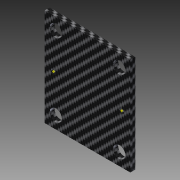
# Autodesk Inventor part: carbon_bump_servo
Saved by Autodesk Inventor 2015 SP1 (Build 190203100, 203)
## iProperties
Created: 2015-07-16
Part Number: carbon_bump_servo
Material: Generic
Document SubType Name: Modeling
Designer: Alexandre Cherpillod
Density: 1 g/cm^3
Appearance: Carbon Fiber
Mass: 2.63035 g
Surface Area: 30.8115 cm^2
Volume: 2.63035 cm^3
Author: Alexandre Cherpillod
Autodesk Inventor part; units mm, degrees
ref_plane "YZ Plane" through (0, 0, 0) normal (1, 0, 0) x (0, 1, 0)
ref_plane "XZ Plane" through (0, 0, 0) normal (0, 1, 0) x (-1, 0, 0)
ref_plane "XY Plane" through (0, 0, 0) normal (0, 0, 1) x (1, 0, 0)
sketch "Sketch1" plane through (0, 0, 0) normal (0, 1, 0) x (-1, 0, 0)
  line L0 (0, 0) -> (35, 0)
  line L1 (35, 0) -> (35, -40)
  line L2 (35, -40) -> (0, -40)
  line L3 (0, -40) -> (0, 0)
  line L4 (35, -40) -> (0, 0) construction
  line L5 (35, 0) -> (0, -40) construction
  line L6 (4.5, -5) -> (30.5, -5) construction
  line L7 (30.5, -5) -> (30.5, -35) construction
  line L8 (30.5, -35) -> (4.5, -35) construction
  line L9 (4.5, -35) -> (4.5, -5) construction
  line L10 (4.5, -5) -> (30.5, -35) construction
  line L11 (30.5, -5) -> (4.5, -35) construction
  circle A0 centre (30.5, -5) radius 2.5
  circle A1 centre (30.5, -35) radius 2.5
  circle A2 centre (4.5, -35) radius 2.5
  circle A3 centre (4.5, -5) radius 2.5
  point P0 (17.5, -20)
  dimension "d0" = 35
  dimension "d1" = 40
  dimension "d2" = 26
  dimension "d3" = 30
  dimension "d4" = 5
  constraints: 24 end point, 4 centre point, 4 coincident, 4 parallel, 3 equal radius, 3 midpoint, 2 horizontal, 2 perpendicular
  measures "d0" distance of L1.end L2.end
  measures "d1" distance of L0.end L1.end
  measures "d2" distance of L7.end L8.end
  measures "d3" distance of L6.end L7.end
  measures "d4" diameter of A0
extrude "Extrusion1" add sketch "Sketch1" along normal blind 2
sketch "Sketch2" plane through (0, 0, 0) normal (0, -1, 0) x (1, 0, 0)
  line L0 (-47.1371, -20) -> (16.7906, -20) construction
  line L1 (-30.5, -5) -> (-4.5, -35) construction
  line L2 (-4.5, -5) -> (-30.5, -35) construction
  point P0 (0, 0)
  point P1 (-17.5, -20)
  point P2 (-17.5, -20)
  point P3 (-31.5, -20)
  point P4 (-3.5, -20)
  dimension "d10" = 14
  dimension "d11" = 14
  constraints: 3 point on line, 2 end point, 2 midpoint, 1 horizontal
  measures "d10" distance of point (-17.5, -20) point (-3.5, -20)
  measures "d11" distance of point (-17.5, -20) point (-31.5, -20)
hole "Hole1" at (-31.5, 0, -20) at (-3.5, 0, -20) direction (0, 1, 0) diameter 2 end through all
body "Solid1"
